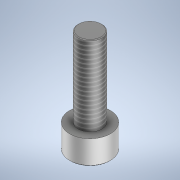
# Autodesk Inventor part: Tornillo allen cabeza cilindrica M6x20mm
Saved by Autodesk Inventor 2020 (Build 240168000, 168)
## iProperties
Created: 2020-05-19
Part Number: Tornillo allen cabeza cilindrica M6x20mm
Material: Genérico
Document SubType Name: Modeling
Designer: Pipi
Density: 1 g/cm^3
Appearance: Goma - Negro - Versión 1.1
Author: Pipi
Autodesk Inventor part; units mm, degrees
ref_plane "YZ Plane" through (0, 0, 0) normal (1, 0, 0) x (0, 1, 0)
ref_plane "XZ Plane" through (0, 0, 0) normal (0, 1, 0) x (-1, 0, 0)
ref_plane "XY Plane" through (0, 0, 0) normal (0, 0, 1) x (1, 0, 0)
sketch "Boceto1" plane through (0, 0, 0) normal (0, 1, 0) x (-1, 0, 0)
  circle A0 centre (8.7689, 12.9363) radius 3
  circle A1 centre (8.7689, 12.9363) radius 5.11
  point P0 (0, 0)
  dimension "d0" = 6
  dimension "d1" = 10.22
  constraints: 2 centre point, 1 coincident
  measures "d0" diameter of A0
  measures "d1" diameter of A1
extrude "Extrusión1" add sketch "Boceto1" along normal blind 20 contours A0
extrude "Extrusión2" add sketch "Boceto1" against normal blind 6 contours A0 | A1
sketch "Boceto2" plane through (-8.7689, -6, 12.9363) normal (0, -1, 0) x (1, 0, 0)
  line L0 (-2.5726, -1.4793) -> (-2.5674, 1.4883)
  line L1 (-2.5674, 1.4883) -> (0.0052, 2.9676)
  line L2 (0.0052, 2.9676) -> (2.5726, 1.4793)
  line L3 (2.5726, 1.4793) -> (2.5674, -1.4883)
  line L4 (2.5674, -1.4883) -> (-0.0052, -2.9676)
  line L5 (-0.0052, -2.9676) -> (-2.5726, -1.4793)
  point P0 (8.7689, -12.9363)
  point P1 (0, 0)
  dimension "d6" = 5.14
  constraints: 12 end point, 13 other
  measures "d6" distance between parallel lines of L5 L2
extrude "Extrusión3" cut sketch "Boceto2" against normal blind 3
thread "Rosca1" size "M6x1" class "6g" standard "ISO Metric profile" length 430
chamfer "Chaflán1" distance 0.2 angle 45 1 edges at (-3.6589, -6, 12.9363) measured on face at (-12.1856, -6, 12.9393)
chamfer "Chaflán2" distance 0.2 angle 45 1 edges at (-5.7689, 20, 12.9363) measured on face at (-7.9784, 20, 13.0158)
